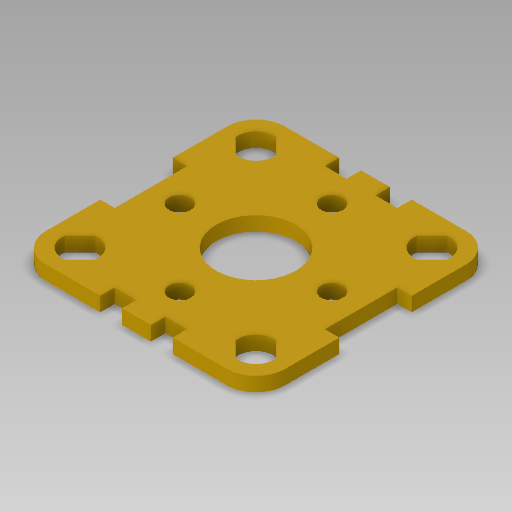
# Autodesk Inventor part: Base1
Saved by Autodesk Inventor 2020 (Build 240168000, 168)
## iProperties
Created: 2019-04-28
Part Number: Base1
Material: Generic
Document SubType Name: Modeling
Designer: Plo
Density: 1 g/cm^3
Appearance: Gold
Author: Plo
Autodesk Inventor part; units mm, degrees
ref_plane "YZ Plane" through (0, 0, 0) normal (1, 0, 0) x (0, 1, 0)
ref_plane "XZ Plane" through (0, 0, 0) normal (0, 1, 0) x (-1, 0, 0)
ref_plane "XY Plane" through (0, 0, 0) normal (0, 0, 1) x (1, 0, 0)
sketch "Sketch1" plane through (0, 0, 0) normal (0, 1, 0) x (-1, 0, 0)
  line L0 (16.5, 12.5) -> (16.5, 6.5)
  line L1 (16.5, -12.5) -> (16.5, -6.5)
  line L2 (16.5, 5) -> (14.5, 5)
  line L3 (14.5, 5) -> (14.5, -5)
  line L4 (5, -16.5) -> (5, -14.5)
  line L5 (-16.5, -5) -> (-14.5, -5)
  line L6 (-14.5, -5) -> (-14.5, 5)
  line L7 (-5, 16.5) -> (-5, 14.5)
  line L8 (5, 14.5) -> (5, 16.5)
  line L9 (16.5, 5) -> (14.5, 5)
  line L10 (16.5, -5) -> (14.5, -5)
  line L11 (5, -16.5) -> (5, -14.5)
  line L12 (-5, -16.5) -> (-5, -14.5)
  line L13 (-5, 14.5) -> (-5, 16.5)
  line L14 (-14.5, 5) -> (-16.5, 5)
  line L15 (-14.5, -5) -> (-16.5, -5)
  line L16 (16.5, 12.5) -> (16.5, 5)
  line L17 (16.5, -5) -> (16.5, -12.5)
  line L18 (12.5, -16.5) -> (5, -16.5)
  line L19 (-5, -16.5) -> (-12.5, -16.5)
  line L20 (-12.5, 16.5) -> (-5, 16.5)
  line L21 (5, 16.5) -> (12.5, 16.5)
  line L22 (-16.5, -12.5) -> (-16.5, -5)
  line L23 (-16.5, 5) -> (-16.5, 12.5)
  arc A0 (12.5, -16.5) -> (16.5, -12.5) centre (12.5, -12.5) ccw
  arc A1 (-16.5, -12.5) -> (-12.5, -16.5) centre (-12.5, -12.5) ccw
  arc A2 (-12.5, 16.5) -> (-16.5, 12.5) centre (-12.5, 12.5) ccw
  arc A3 (16.5, 12.5) -> (12.5, 16.5) centre (12.5, 12.5) ccw
  line L24 (14.5, 0) -> (10.5, 0)
  circle A4 centre (10.5, 0) radius 1.5
  line L25 (-14.5, 0) -> (-10.5, 0)
  circle A5 centre (-10.5, 0) radius 1.5
  circle A6 centre (0, 10.5) radius 1.5
  circle A7 centre (0, -10.5) radius 1.5
  circle A8 centre (0, 0) radius 5.5
  line L26 (2, -14.5) -> (2, -16.5)
  line L27 (2, -16.5) -> (-2, -16.5)
  line L28 (-2, -16.5) -> (-2, -14.5)
  line L29 (0, 16.5) -> (2, 16.5)
  line L30 (2, 16.5) -> (2, 14.5)
  line L31 (5, -14.5) -> (2, -14.5)
  line L32 (-2, -14.5) -> (-5, -14.5)
  line L33 (0, 16.5) -> (-2, 16.5)
  line L34 (-2, 16.5) -> (-2, 14.5)
  line L35 (-5, 14.5) -> (-2, 14.5)
  line L36 (2, 14.5) -> (5, 14.5)
  line L37 (16.5, 16.5) -> (15.3284, 15.3284) construction
  line L38 (13.9142, 13.9142) -> (-16.5, -16.5) construction
  line L39 (13.5607, 10.7322) -> (12.5, 9.6716)
  line L40 (13.5607, 10.7322) -> (14.6213, 11.7929)
  line L41 (10.7322, 13.5607) -> (9.6716, 12.5)
  line L42 (10.7322, 13.5607) -> (11.7929, 14.6213)
  arc A9 (14.6213, 11.7929) -> (11.7929, 14.6213) centre (12.1464, 12.1464) ccw
  arc A10 (9.6716, 12.5) -> (12.5, 9.6716) centre (12.1464, 12.1464) ccw
  line L43 (13.5607, -10.7322) -> (12.5, -9.6716)
  line L44 (13.5607, -10.7322) -> (14.6213, -11.7929)
  line L45 (10.7322, -13.5607) -> (11.7929, -14.6213)
  line L46 (10.7322, -13.5607) -> (9.6716, -12.5)
  arc A11 (11.7929, -14.6213) -> (14.6213, -11.7929) centre (12.1464, -12.1464) ccw
  arc A12 (12.5, -9.6716) -> (9.6716, -12.5) centre (12.1464, -12.1464) ccw
  line L47 (0, 16.5) -> (0, 14.5)
  line L48 (-13.5607, 10.7322) -> (-12.5, 9.6716)
  line L49 (-13.5607, 10.7322) -> (-14.6213, 11.7929)
  line L50 (-10.7322, 13.5607) -> (-11.7929, 14.6213)
  line L51 (-10.7322, 13.5607) -> (-9.6716, 12.5)
  arc A13 (-11.7929, 14.6213) -> (-14.6213, 11.7929) centre (-12.1464, 12.1464) ccw
  arc A14 (-12.5, 9.6716) -> (-9.6716, 12.5) centre (-12.1464, 12.1464) ccw
  line L52 (-13.5607, -10.7322) -> (-14.6213, -11.7929)
  arc A15 (-14.6213, -11.7929) -> (-11.7929, -14.6213) centre (-12.1464, -12.1464) ccw
  arc A16 (-9.6716, -12.5) -> (-12.5, -9.6716) centre (-12.1464, -12.1464) ccw
  line L53 (-10.7322, -13.5607) -> (-9.6716, -12.5)
  line L54 (-13.5607, -10.7322) -> (-12.5, -9.6716)
  line L55 (-10.7322, -13.5607) -> (-11.7929, -14.6213)
  point P0 (-16.5, 16.5)
  point P1 (16.5, -16.5)
  dimension "d0" = 33
  dimension "d1" = 33
  dimension "d18" = 4
  dimension "d19" = 4
  dimension "d20" = 4
  dimension "d21" = 4
  dimension "d23" = 3
  constraints: 112 end point, 33 perpendicular, 27 point on circle, 24 symmetric about line, 17 centre point, 11 point on line, 8 parallel, 8 tangent, 5 horizontal, 2 coincident, 2 midpoint, 1 vertical, 6 other
  measures "d0" distance of point (16.5, -16.5) L38.end
  measures "d1" distance of L37.start point (16.5, -16.5)
  measures "d18" radius of A0
  measures "d19" radius of A1
  measures "d20" radius of A2
  measures "d21" radius of A3
  measures "d23" diameter of A4
extrude "Extrusion2" add sketch "Sketch1" along normal blind 2
body "Solid2"
